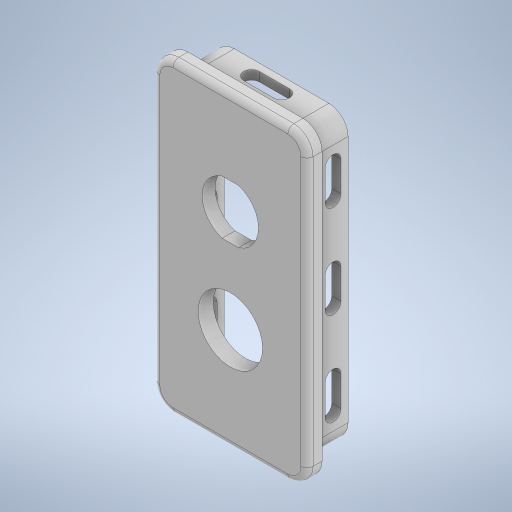
# Autodesk Inventor part: 2x4_Endcap
Saved by Autodesk Inventor 2023 (Build 270158000, 158)
## iProperties
Created: 2023-06-19
Part Number: 2x4_Endcap
Material: Generic
Document SubType Name: Modeling
Designer: plebbb
Density: 1 g/cm^3
Appearance: Default
Author: plebbb
Autodesk Inventor part; units mm, degrees
ref_plane "YZ Plane" through (0, 0, 0) normal (1, 0, 0) x (0, 1, 0)
ref_plane "XZ Plane" through (0, 0, 0) normal (0, 1, 0) x (-1, 0, 0)
ref_plane "XY Plane" through (0, 0, 0) normal (0, 0, 1) x (1, 0, 0)
sketch "Sketch1" plane through (0, 0, 0) normal (0, 0, 1) x (1, 0, 0)
  line L0 (6.35, 0) -> (44.45, 0)
  line L1 (50.8, 6.35) -> (50.8, 95.25)
  line L2 (44.45, 101.6) -> (6.35, 101.6)
  line L3 (0, 95.25) -> (0, 6.35)
  arc A0 (6.35, 101.6) -> (0, 95.25) centre (6.35, 95.25) ccw
  arc A1 (0, 6.35) -> (6.35, 0) centre (6.35, 6.35) ccw
  arc A2 (44.45, 0) -> (50.8, 6.35) centre (44.45, 6.35) ccw
  arc A3 (50.8, 95.25) -> (44.45, 101.6) centre (44.45, 95.25) ccw
  point P0 (0, 0)
  point P1 (50.8, 101.6)
  point P2 (50.8, 0)
  point P3 (0, 101.6)
  dimension "d0" = 101.6
  dimension "d1" = 50.8
  dimension "d2" = 6.35
  constraints: 8 end point, 8 point on circle, 8 point on line, 8 tangent, 4 centre point, 3 equal radius, 2 parallel, 1 horizontal, 1 perpendicular
  measures "d0" distance of point (50.8, 0) point (50.8, 101.6)
  measures "d1" distance of point (50.8, 101.6) point (0, 101.6)
  measures "d2" radius of A0
extrude "Extrusion1" add sketch "Sketch1" along normal blind 5
fillet "Fillet1" radius 2 8 edges at (1.8599, 99.7401, 5) (0, 50.8, 5) (1.8599, 1.8599, 5) (25.4, 0, 5) (48.9401, 1.8599, 5) (50.8, 50.8, 5) (48.9401, 99.7401, 5) (25.4, 101.6, 5)
sketch "Sketch3" plane through (0, 0, 0) normal (0, 0, -1) x (-1, 0, 0)
  circle A0 centre (-25.4, 33.8667) radius 10.6775
  line L0 (-6.35, 0) -> (-44.45, 0) construction
  line L1 (-44.45, 101.6) -> (-6.35, 101.6) construction
  line L2 (-25.4, 101.6) -> (-25.4, 0) construction
  line L3 (-17.4326, 20.0667) -> (-33.3674, 20.0667)
  line L4 (-33.3674, 20.0667) -> (-41.3349, 33.8667)
  line L5 (-41.3349, 33.8667) -> (-33.3674, 47.6667)
  line L6 (-33.3674, 47.6667) -> (-17.4326, 47.6667)
  line L7 (-17.4326, 47.6667) -> (-9.4651, 33.8667)
  line L8 (-9.4651, 33.8667) -> (-17.4326, 20.0667)
  point P0 (0, 0)
  point P1 (-25.4, 33.8667)
  dimension "d8" = 21.355
  dimension "d9" = 33.8667
  dimension "d20" = 27.6
  constraints: 14 end point, 3 midpoint, 1 centre point, 1 coincident, 1 horizontal, 1 point on line, 13 other
  measures "d8" diameter of A0
  measures "d9" distance of point (-25.4, 0) A0.centre
  measures "d20" distance between parallel lines of L6 L3
sketch "Sketch2" plane through (0, 0, 0) normal (0, 0, -1) x (-1, 0, 0)
  line L0 (-41.075, 3.375) -> (-9.725, 3.375)
  line L1 (-3.375, 9.725) -> (-3.375, 91.875)
  line L2 (-9.725, 98.225) -> (-41.075, 98.225)
  line L3 (-47.425, 91.875) -> (-47.425, 9.725)
  line L4 (-44.45, 101.6) -> (-6.35, 101.6) construction
  line L5 (-50.8, 6.35) -> (-50.8, 95.25) projected
  line L6 (-25.4, 98.225) -> (-25.4, 101.6) construction
  line L7 (-50.8, 6.35) -> (-50.8, 95.25) construction
  line L8 (-50.8, 50.8) -> (-47.425, 50.8) construction
  arc A0 (-41.075, 98.225) -> (-47.425, 91.875) centre (-41.075, 91.875) ccw
  arc A1 (-3.375, 91.875) -> (-9.725, 98.225) centre (-9.725, 91.875) ccw
  arc A2 (-47.425, 9.725) -> (-41.075, 3.375) centre (-41.075, 9.725) ccw
  arc A3 (-9.725, 3.375) -> (-3.375, 9.725) centre (-9.725, 9.725) ccw
  arc A4 (-44.425, 9.725) -> (-41.075, 6.375) centre (-41.075, 9.725) ccw
  arc A5 (-9.725, 6.375) -> (-6.375, 9.725) centre (-9.725, 9.725) ccw
  arc A6 (-6.375, 91.875) -> (-9.725, 95.225) centre (-9.725, 91.875) ccw
  arc A7 (-41.075, 95.225) -> (-44.425, 91.875) centre (-41.075, 91.875) ccw
  line L9 (-44.425, 91.875) -> (-44.425, 9.725)
  line L10 (-48.8, 95.25) -> (-48.8, 6.35) projected
  line L11 (-41.075, 6.375) -> (-9.725, 6.375)
  line L12 (-6.375, 9.725) -> (-6.375, 91.875)
  line L13 (-9.725, 95.225) -> (-41.075, 95.225)
  point P0 (0, 0)
  point P1 (-9.725, 6.375)
  dimension "d6" = 3.375
  dimension "d7" = 6.35
  dimension "d14" = 3
  dimension "d15" = 3
  constraints: 20 end point, 16 point on circle, 10 tangent, 8 centre point, 6 equal radius, 5 midpoint, 4 coincident, 4 perpendicular, 3 equal length, 3 parallel, 2 horizontal, 1 vertical
  measures "d6" distance of L8.start L8.end
  measures "d7" radius of A0
  measures "d14" distance between parallel lines of L2 L13
  measures "d15" distance between parallel lines of L1 L12
sketch "Sketch4" plane through (0, 0, 0) normal (0, 0, -1) x (-1, 0, 0)
  line L0 (-25.4, 101.6) -> (-25.4, 0) construction
  circle A0 centre (-25.4, 67.7333) radius 9.325
  line L1 (-44.45, 101.6) -> (-6.35, 101.6) construction
  line L2 (-28.1019, 76.6583) -> (-22.6981, 76.6583)
  line L3 (-22.6981, 58.8083) -> (-28.1019, 58.8083)
  point P0 (0, 0)
  dimension "d10" = 33.8667
  dimension "d11" = 18.65
  dimension "d13" = 17.85
  constraints: 4 end point, 4 point on circle, 2 parallel, 1 centre point, 1 horizontal, 1 point on line
  measures "d10" distance from line of A0.centre L1
  measures "d11" diameter of A0
  measures "d13" distance between parallel lines of L3 L2
extrude "Extrusion2" add sketch "Sketch2" along normal blind 12
extrude "Extrusion3" cut sketch "Sketch4" against normal up to surface (5 mm away) contours A0 L3 L2
extrude "Extrusion4" cut sketch "Sketch3" against normal up to surface (5 mm away) contours A0
sketch "Sketch5" plane through (0, 0, 0) normal (0, 0, -1) x (-1, 0, 0)
  arc A0 (-28.1019, 76.6583) -> (-28.1019, 58.8083) centre (-25.4, 67.7333) ccw projected
  circle A1 centre (-25.4, 67.7333) radius 10.875
  point P0 (0, 0)
  dimension "d23" = 21.75
  constraints: 1 centre point, 1 coincident
  measures "d23" diameter of A1
extrude "Extrusion5" cut sketch "Sketch5" against normal blind 0.75
chamfer "Chamfer1" distance 3 angle 45 8 edges at (6.375, 50.8, 0) (7.3562, 94.2438, 0) (25.4, 95.225, 0) (43.4438, 94.2438, 0) (44.425, 50.8, 0) (43.4438, 7.3562, 0) (25.4, 6.375, 0) (7.3562, 7.3562, 0)
sketch "Sketch6" plane through (47.425, 9.725, 0) normal (1, 0, 0) x (0, 0, -1)
  line L0 (7, 15.275) -> (7, 5.275) construction
  line L1 (9.613, 15.275) -> (9.613, 5.275)
  line L2 (4.387, 5.275) -> (4.387, 15.275)
  arc A0 (9.613, 15.275) -> (4.387, 15.275) centre (7, 15.275) ccw
  arc A1 (4.387, 5.275) -> (9.613, 5.275) centre (7, 5.275) ccw
  line L3 (0, -9.725) -> (7, -9.725) construction
  line L4 (7, -9.725) -> (7, 91.875) construction
  line L5 (0, 91.875) -> (0, 85.525) construction
  line L6 (0, 91.875) -> (7, 91.875) construction
  line L7 (7, 76.875) -> (7, 66.875) construction
  line L8 (9.613, 76.875) -> (9.613, 66.875)
  line L9 (4.387, 66.875) -> (4.387, 76.875)
  arc A2 (9.613, 76.875) -> (4.387, 76.875) centre (7, 76.875) ccw
  arc A3 (4.387, 66.875) -> (9.613, 66.875) centre (7, 66.875) ccw
  line L10 (7, 46.075) -> (7, 36.075) construction
  line L11 (9.613, 46.075) -> (9.613, 36.075)
  line L12 (4.387, 36.075) -> (4.387, 46.075)
  arc A4 (9.613, 46.075) -> (4.387, 46.075) centre (7, 46.075) ccw
  arc A5 (4.387, 36.075) -> (9.613, 36.075) centre (7, 36.075) ccw
  point P0 (7, 10.275)
  point P1 (7, 71.875)
  point P2 (7, 41.075)
  dimension "d29" = 2.613
  dimension "d30" = 7
  dimension "d31" = 2.613
  dimension "d32" = 20
  dimension "d33" = 20
  dimension "d34" = 2.613
  dimension "d35" = 10
  constraints: 30 end point, 12 point on circle, 12 tangent, 6 centre point, 5 midpoint, 3 parallel, 3 vertical, 2 collinear, 2 perpendicular, 2 point on line, 1 horizontal
  measures "d29" radius of A1
  measures "d30" distance of L3.start L3.end
  measures "d31" radius of A3
  measures "d32" distance from line of L3 point (7, 10.275)
  measures "d33" distance of L4.end point (7, 71.875)
  measures "d34" radius of A5
  measures "d35" distance of L2.start L2.end
extrude "Extrusion6" cut sketch "Sketch6" against normal through all
sketch "Sketch7" plane through (9.725, 98.225, 0) normal (0, 1, 0) x (1, 0, 0)
  line L0 (-9.725, 0) -> (-9.725, -3) construction
  line L1 (-9.725, 0) -> (-9.725, 7) construction
  line L2 (-9.725, 7) -> (41.075, 7) construction
  line L3 (41.075, 7) -> (41.075, 0) construction
  line L4 (10.675, 7) -> (20.675, 7) construction
  line L5 (10.675, 4.387) -> (20.675, 4.387)
  line L6 (20.675, 9.613) -> (10.675, 9.613)
  arc A0 (10.675, 9.613) -> (10.675, 4.387) centre (10.675, 7) ccw
  arc A1 (20.675, 4.387) -> (20.675, 9.613) centre (20.675, 7) ccw
  point P0 (15.675, 7)
  dimension "d38" = 2.613
  dimension "d39" = 10
  dimension "d40" = 7
  constraints: 14 end point, 4 point on circle, 4 tangent, 2 centre point, 2 midpoint, 2 perpendicular, 1 coincident, 1 collinear, 1 parallel, 1 vertical
  measures "d38" radius of A1
  measures "d39" distance of L6.start L6.end
  measures "d40" distance of L2.end L3.end
extrude "Extrusion7" cut sketch "Sketch7" against normal through all
body "Solid1"
